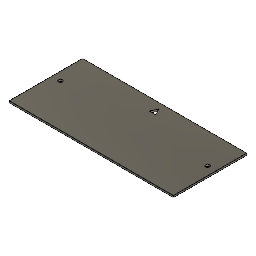
smmb_inner-top (Autodesk Fusion 360 design; units mm, degrees)
Autodesk Fusion 360 part; units mm, degrees
sketch "Sketch1" plane through (0, 0, 0) normal (0, 0, 1) x (1, 0, 0)
  line L0 (0, 0) -> (134, 0)
  line L1 (134, 0) -> (134, 60)
  line L2 (134, 60) -> (0, 60)
  line L3 (0, 60) -> (0, 0)
  circle A0 centre (7, 35) radius 1.55
  line L4 (67, 0) -> (67, 60) construction
  circle A1 centre (127, 35) radius 1.55
  line L5 (69.5, 50) -> (64.5, 50)
  line L6 (64.5, 50) -> (64.5, 55)
  line L7 (64.5, 55) -> (69.5, 55)
  line L8 (69.5, 55) -> (69.5, 50)
  line L9 (69.5, 50) -> (64.5, 55) construction
  line L10 (64.5, 50) -> (69.5, 55) construction
  line L11 (64.5, 50) -> (67, 55)
  line L12 (67, 55) -> (69.5, 50)
  point P0 (67, 52.5)
  dimension "d1" = 134
  dimension "d2" = 60
  dimension "d3" = 3.1
  dimension "d4" = 7
  dimension "d5" = 25
  dimension "d6" = 5
  dimension "d7" = 5
  dimension "d8" = 5
  constraint horizontal L0
  constraint vertical L1
  constraint horizontal L2
  constraint vertical L3
  constraint coincident L0.start L3.end
  constraint midpoint L0 L4.start
  constraint midpoint L2 L4.end
  constraint symmetric A0 L4 A1
  constraint perpendicular L5 L6
  constraint parallel L5 L7
  constraint parallel L6 L8
  constraint horizontal L5
  constraint coincident L9 P0
  constraint coincident L10 P0
  constraint coincident L4 P0
  constraint midpoint L7 L11.end
  measures "d1" distance of L0.start L0.end
  measures "d2" distance of L0.start L2.end
  measures "d3" diameter of A0
  measures "d4" distance of L3 A0.centre
  measures "d5" distance of L2 A0.centre
  measures "d6" distance of L5.end L6.end
  measures "d7" distance of L6.end L7.end
  measures "d8" distance of L2 L7
extrude "Extrude1" add sketch "Sketch1" along normal blind 1.5 contours L0 L1 L2 L3 | L7 L8 L12 | L6 L7 L11
